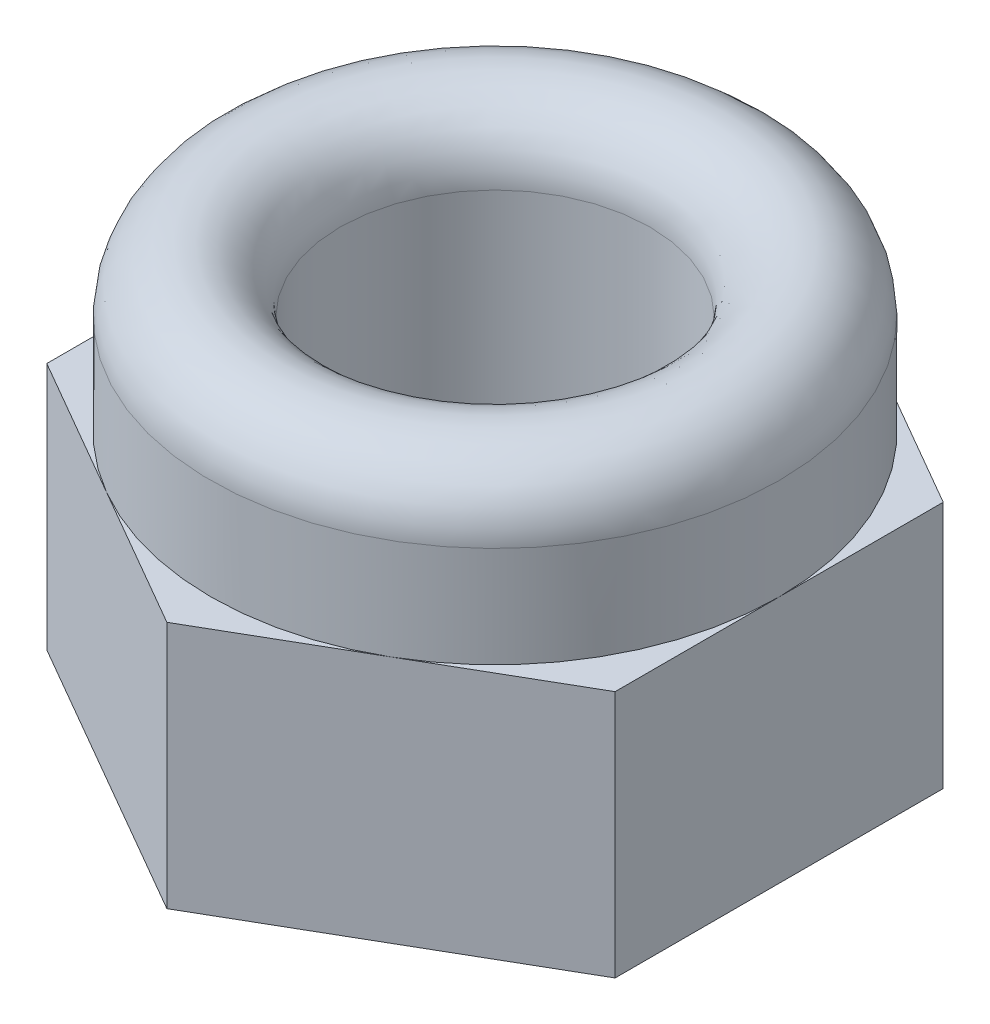
# Autodesk Inventor part: m3LockNute
Saved by Autodesk Inventor 2023 (Build 270158000, 158)
## iProperties
Created: 2022-09-11
Part Number: m3LockNute
Material: Generic
Document SubType Name: Modeling
Designer: deli
Density: 1 g/cm^3
Appearance: Default
Author: deli
Autodesk Inventor part; units mm, degrees
ref_plane "YZ Plane" through (0, 0, 0) normal (1, 0, 0) x (0, 1, 0)
ref_plane "XZ Plane" through (0, 0, 0) normal (0, 1, 0) x (-1, 0, 0)
ref_plane "XY Plane" through (0, 0, 0) normal (0, 0, 1) x (1, 0, 0)
sketch "Sketch1" plane through (0, 0, 0) normal (0, 1, 0) x (-1, 0, 0)
  line L0 (38.5716, -36.1268) -> (41.3216, -34.5391)
  line L1 (41.3216, -34.5391) -> (44.0716, -36.1268)
  line L2 (44.0716, -36.1268) -> (44.0716, -39.3022)
  line L3 (44.0716, -39.3022) -> (41.3216, -40.8899)
  line L4 (41.3216, -40.8899) -> (38.5716, -39.3022)
  line L5 (38.5716, -39.3022) -> (38.5716, -36.1268)
  circle A0 centre (41.3216, -37.7145) radius 1.5
  point P0 (0, 0)
  dimension "d0" = 5.5
  dimension "d1" = 3
  constraints: 12 end point, 1 centre point, 1 coincident, 1 vertical, 13 other
  measures "d0" distance between parallel lines of L5 L2
  measures "d1" diameter of A0
extrude "Extrusion1" add sketch "Sketch1" along normal blind 2.4
sketch "Sketch2" plane through (0, 2.4, 0) normal (0, 1, 0) x (1, 0, 0)
  circle A0 centre (-41.3216, 37.7145) radius 1.5 projected
  circle A1 centre (-41.3216, 37.7145) radius 2.75
  line L0 (-44.0716, 39.3022) -> (-44.0716, 36.1268) projected
  point P0 (0, 0)
  constraints: 1 centre point, 1 coincident, 1 tangent
extrude "Extrusion2" add sketch "Sketch2" along normal blind 1.6
fillet "Fillet1" radius 0.625 2 edges at (-44.0716, 4, -37.7145) (-42.8216, 4, -37.7145)
body "Solid1"
